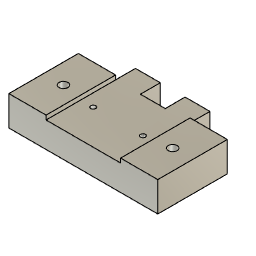
motor_mount_spacer_plate v51 (Autodesk Fusion 360 design; units mm, degrees)
Autodesk Fusion 360 part; units mm, degrees
sketch "Sketch1" plane through (0, 0, 0) normal (0, 0, 1) x (1, 0, 0)
  line L0 (0, 0) -> (57, 0)
  line L1 (57, 0) -> (57, 30)
  line L2 (57, 30) -> (0, 30)
  line L3 (0, 30) -> (0, 0)
  dimension "d1" = 57
  dimension "d2" = 30
  constraint horizontal L0
  constraint vertical L1
  constraint horizontal L2
  constraint vertical L3
  constraint coincident L0.start L3.end
  measures "d1" distance of L0.start L0.end
  measures "d2" distance of L0.start L2.end
extrude "Extrude1" add sketch "Sketch1" along normal blind 20.719
extrude "Extrude2" add 1 faces at (19, 20, 20.719) along direction (0, 0, 1) blind 10.719
extrude "Extrude3" add 1 faces at (19, 0, 10.4793) along direction (0, -1, 0) blind 10
extrude "Extrude4" cut 1 faces at (19, -10, 10.4793) along direction (0, 1, 0) blind 2
sketch "Sketch2" plane through (0, 0, 31.438) normal (0, 0, 1) x (-1, 0, 0)
  line L0 (0, 8) -> (-57, 8)
  line L1 (-57, 8) -> (-57, -30)
  line L2 (-57, -30) -> (0, -30)
  line L3 (0, -30) -> (0, 8)
  line L4 (0, -30) -> (0, -11)
  line L5 (0, -11) -> (-14.754, -11)
  line L6 (-57, -11) -> (-42.246, -11)
  dimension "d11" = 19
  dimension "d12" = 14.754
  dimension "d13" = 14.754
  constraint coincident L2.end L3.start
  constraint perpendicular L0 L4
  constraint perpendicular L4 L5
  constraint midpoint L1 L6.start
  constraint perpendicular L1 L6
  measures "d11" distance of L2.end L4.end
  measures "d12" distance of L4.end L5.end
  measures "d13" distance of L6.start L6.end
hole "Hole1" at (14.754, 11, 31.438) at (42.246, 11, 31.438) direction (0, 0, -1) diameter 6.6 depth 50 tip angle 180
sketch "Sketch3" plane through (0, 0, 31.438) normal (0, 0, 1) x (-1, 0, 0)
  circle A0 centre (-14.754, -11) radius 3.3
  circle A1 centre (-42.246, -11) radius 3.3
  line L0 (0, 8) -> (-57, 8)
  line L1 (-57, 8) -> (-57, -30)
  line L2 (-57, -30) -> (0, -30)
  line L3 (0, -30) -> (0, 8)
  line L4 (-14.754, -11) -> (-14.754, 0.251)
  line L5 (-42.246, -11) -> (-42.246, 0.251)
  dimension "d17" = 11.251
  dimension "d18" = 11.251
  constraint coincident A0.centre L4.start
  constraint vertical L4
  constraint coincident A1.centre L5.start
  constraint vertical L5
  measures "d17" distance of A0.centre L4.end
  measures "d18" distance of A1.centre L5.end
hole "Hole2" at (14.754, -0.251, 31.438) at (42.246, -0.251, 31.438) direction (0, 0, -1) diameter 6.6 depth 50 tip angle 180
delete_face "DeleteFace1" 1 faces at (15.0826, 7.7164, 20.9587)
delete_face "DeleteFace2" 1 faces at (42.5746, 7.7164, 20.9587)
delete_face "DeleteFace3" 1 faces at (15.0826, -3.5346, 20.9587)
delete_face "DeleteFace4" 1 faces at (42.5746, -3.5346, 20.9587)
sketch "Sketch4" plane through (0, 0, 31.438) normal (0, 0, 1) x (-1, 0, 0)
  line L0 (0, 8) -> (-57, 8)
  line L1 (-57, 8) -> (-57, -30)
  line L2 (-57, -30) -> (0, -30)
  line L3 (0, -30) -> (0, 8)
  line L4 (0, 8) -> (-14.754, 8)
  line L5 (-14.754, 8) -> (-14.754, -2)
  line L6 (-14.754, -2) -> (0, -2)
  line L7 (0, -2) -> (0, 8)
  line L8 (-57, 8) -> (-42.246, 8)
  line L9 (-42.246, 8) -> (-42.246, -2)
  line L10 (-42.246, -2) -> (-57, -2)
  line L11 (-57, -2) -> (-57, 8)
  dimension "d22" = 14.754
  dimension "d23" = 10
  dimension "d24" = 14.754
  dimension "d25" = 10
  constraint horizontal L4
  constraint vertical L5
  constraint horizontal L6
  constraint vertical L7
  constraint coincident L0.start L3.end
  constraint horizontal L8
  constraint vertical L9
  constraint horizontal L10
  constraint vertical L11
  constraint coincident L0.end L1.start
  measures "d22" distance of L0.start L4.end
  measures "d23" distance of L0.start L6.end
  measures "d24" distance of L0.end L8.end
  measures "d25" distance of L0.end L10.end
hole "Hole3" at (14.754, 2, 31.438) at (42.246, 2, 31.438) direction (0, 0, -1) diameter 6.6 depth 48 tip angle 180
delete_face "DeleteFace5" 1 faces at (15.0826, -1.2836, 20.9587)
delete_face "DeleteFace6" 1 faces at (42.5746, -1.2836, 20.9587)
sketch "Sketch5" plane through (0, 0, 31.438) normal (0, 0, 1) x (-1, 0, 0)
  line L0 (0, 8) -> (-57, 8)
  line L1 (-57, 8) -> (-57, -30)
  line L2 (-57, -30) -> (0, -30)
  line L3 (0, -30) -> (0, 8)
  line L4 (0, 8) -> (-28.5, 8)
  line L5 (-28.5, 8) -> (-28.5, -11)
  line L6 (-28.5, -11) -> (0, -11)
  line L7 (0, -11) -> (0, 8)
  line L8 (-28.5, -11) -> (-14.754, -11)
  line L9 (-14.754, -11) -> (-14.754, 2.746)
  line L10 (-14.754, 2.746) -> (-28.5, 2.746)
  line L11 (-28.5, 2.746) -> (-28.5, -11)
  line L12 (-14.754, 2.746) -> (-42.246, 2.746)
  line L13 (-42.246, 2.746) -> (-42.246, -24.746)
  line L14 (-42.246, -24.746) -> (-14.754, -24.746)
  line L15 (-14.754, -24.746) -> (-14.754, 2.746)
  dimension "d29" = 28.5
  dimension "d30" = 19
  dimension "d31" = 13.746
  dimension "d32" = 13.746
  dimension "d33" = 27.492
  dimension "d34" = 27.492
  constraint horizontal L4
  constraint vertical L5
  constraint horizontal L6
  constraint vertical L7
  constraint coincident L0.start L3.end
  constraint horizontal L8
  constraint vertical L9
  constraint horizontal L10
  constraint vertical L11
  constraint horizontal L12
  constraint vertical L13
  constraint horizontal L14
  constraint vertical L15
  measures "d29" distance of L0.start L4.end
  measures "d30" distance of L0.start L6.end
  measures "d31" distance of L5.end L8.end
  measures "d32" distance of L5.end L10.end
  measures "d33" distance of L9.end L12.end
  measures "d34" distance of L9.end L14.end
extrude "Extrude5" add 1 faces at (19, -8, 10.4793) along direction (0, -1, 0) blind 1
extrude "Extrude6" add 1 faces at (38, 30, 10.4793) along direction (0, 1, 0) blind 1
sketch "Sketch6" plane through (0, 0, 31.438) normal (0, 0, 1) x (-1, 0, 0)
  line L0 (-57, 9) -> (-57, -31)
  line L1 (-57, -31) -> (0, -31)
  line L2 (0, -31) -> (0, 9)
  line L3 (0, 9) -> (-57, 9)
  line L4 (0, -31) -> (-20, -31)
  line L5 (-20, -31) -> (-20, -41)
  line L6 (-20, -41) -> (0, -41)
  line L7 (0, -41) -> (0, -31)
  line L8 (-57, -31) -> (-37, -31)
  line L9 (-37, -31) -> (-37, -41)
  line L10 (-37, -41) -> (-57, -41)
  line L11 (-57, -41) -> (-57, -31)
  dimension "d42" = 20
  dimension "d43" = 10
  dimension "d44" = 20
  dimension "d45" = 10
  constraint horizontal L4
  constraint vertical L5
  constraint horizontal L6
  constraint vertical L7
  constraint coincident L1.end L2.start
  constraint horizontal L8
  constraint vertical L9
  constraint horizontal L10
  constraint vertical L11
  constraint coincident L0.end L1.start
  measures "d42" distance of L1.end L4.end
  measures "d43" distance of L1.end L6.end
  measures "d44" distance of L0.end L8.end
  measures "d45" distance of L0.end L10.end
extrude "Extrude7" add sketch "Sketch6" against normal up to surface (31.438 mm away) contours L1 L8 L9 L10 L11 | L1 L4 L5 L6 L7
extrude "Extrude8" add 2 faces at (13.3333, 41, 20.9587) (43.6667, 41, 20.9587) along direction (0, 1, 0) blind 10
extrude "Extrude9" cut 1 faces at (31.3333, 4.3333, 31.438) along direction (0, 0, -1) blind 5.719
extrude "Extrude10" add 1 faces at (0, 11, 17.146) along direction (-1, 0, 0) blind 1.25
extrude "Extrude11" add 1 faces at (57, 11, 17.146) along direction (1, 0, 0) blind 1.25
extrude "Extrude12" add 1 faces at (58.25, 11, 17.146) along direction (1, 0, 0) blind 0.25
extrude "Extrude13" add 1 faces at (-1.25, 11, 17.146) along direction (-1, 0, 0) blind 0.25
extrude "Extrude14" cut 1 faces at (20, 37.6667, 17.146) along direction (-1, 0, 0) blind 1.5
extrude "Extrude15" cut 1 faces at (37, 37.6667, 17.146) along direction (1, 0, 0) blind 1.5
sketch "Sketch8" plane through (0, 0, 25.719) normal (0, 0, 1) x (-1, 0, 0)
  line L0 (-38.5, -51) -> (-38.5, -31)
  line L1 (-38.5, -31) -> (-18.5, -31)
  line L2 (-18.5, -31) -> (-18.5, -51)
  line L3 (-18.5, -51) -> (1.5, -51)
  line L4 (1.5, -51) -> (1.5, 9)
  line L5 (1.5, 9) -> (-58.5, 9)
  line L6 (-58.5, 9) -> (-58.5, -51)
  line L7 (-58.5, -51) -> (-38.5, -51)
  line L8 (-28.5, -31) -> (-28.5, -11)
  line L9 (-28.5, -11) -> (-13.5, -11)
  line L10 (-13.5, -11) -> (-13.5, 4)
  line L11 (-13.5, 4) -> (-28.5, 4)
  line L12 (-28.5, 4) -> (-28.5, -11)
  line L13 (-13.5, 4) -> (-43.5, 4)
  line L14 (-43.5, 4) -> (-43.5, -26)
  line L15 (-43.5, -26) -> (-13.5, -26)
  line L16 (-13.5, -26) -> (-13.5, 4)
  dimension "d64" = 15
  dimension "d65" = 15
  dimension "d66" = 30
  dimension "d67" = 30
  constraint midpoint L1 L8.start
  constraint perpendicular L5 L8
  constraint horizontal L9
  constraint vertical L10
  constraint horizontal L11
  constraint vertical L12
  constraint horizontal L13
  constraint vertical L14
  constraint horizontal L15
  constraint vertical L16
  measures "d64" distance of L8.end L9.end
  measures "d65" distance of L8.end L11.end
  measures "d66" distance of L10.end L13.end
  measures "d67" distance of L10.end L15.end
extrude "Extrude16" add 1 faces at (38.5, -9, 8.573) along direction (0, -1, 0) blind 5
extrude "Extrude17" add 2 faces at (11.8333, 51, 17.146) (45.1667, 51, 17.146) along direction (0, 1, 0) blind 5.688
extrude "Extrude18" add 1 faces at (25.1667, 31, 8.573) along direction (0, 1, 0) blind 0.688
extrude "Extrude19" cut 1 faces at (38.5, -14, 8.573) along direction (0, 1, 0) blind 0.788
extrude "Extrude20" add 1 faces at (38.5, -13.212, 8.573) along direction (0, -1, 0) blind 0.1
extrude "Extrude21" cut 1 faces at (18.5, 40.0213, 17.146) along direction (-1, 0, 0) blind 2.5
extrude "Extrude22" cut 1 faces at (38.5, 40.0213, 17.146) along direction (1, 0, 0) blind 2.5
extrude "Extrude23" cut 1 faces at (10.1667, 56.688, 17.146) along direction (0, -1, 0) blind 3
extrude "Extrude24" cut 1 faces at (46.8333, 56.688, 17.146) along direction (0, -1, 0) blind 3
sketch "Sketch9" plane through (0, 0, 25.719) normal (0, 0, 1) x (-1, 0, 0)
  line L0 (-58.5, -53.688) -> (-41, -53.688)
  line L1 (-41, -53.688) -> (-41, -31.688)
  line L2 (-41, -31.688) -> (-16, -31.688)
  line L3 (-16, -31.688) -> (-16, -53.688)
  line L4 (-16, -53.688) -> (1.5, -53.688)
  line L5 (1.5, -53.688) -> (1.5, 13.312)
  line L6 (1.5, 13.312) -> (-58.5, 13.312)
  line L7 (-58.5, 13.312) -> (-58.5, -53.688)
  line L8 (-43.5, -26) -> (-43.5, -23)
  line L9 (-43.5, -23) -> (-13.5, -23)
  line L10 (-13.5, -23) -> (-13.5, 7)
  line L11 (-13.5, 7) -> (-43.5, 7)
  line L12 (-43.5, 7) -> (-43.5, -23)
  dimension "d89" = 3
  dimension "d90" = 30
  dimension "d91" = 30
  constraint vertical L8
  constraint horizontal L9
  constraint vertical L10
  constraint horizontal L11
  constraint vertical L12
  measures "d89" distance of L8.start L8.end
  measures "d90" distance of L8.end L9.end
  measures "d91" distance of L8.end L11.end
sketch "Sketch10" plane through (0, 0, 25.719) normal (0, 0, 1) x (-1, 0, 0)
  line L0 (-58.5, -53.688) -> (-41, -53.688)
  line L1 (-41, -53.688) -> (-41, -31.688)
  line L2 (-41, -31.688) -> (-16, -31.688)
  line L3 (-16, -31.688) -> (-16, -53.688)
  line L4 (-16, -53.688) -> (1.5, -53.688)
  line L5 (1.5, -53.688) -> (1.5, 13.312)
  line L6 (1.5, 13.312) -> (-58.5, 13.312)
  line L7 (-58.5, 13.312) -> (-58.5, -53.688)
  line L8 (-43.5, 7) -> (-43.5, 6.312)
  line L9 (-43.5, 6.312) -> (-13.5, 6.312)
  line L10 (-13.5, 6.312) -> (-13.5, -23.688)
  line L11 (-13.5, -23.688) -> (-43.5, -23.688)
  line L12 (-43.5, -23.688) -> (-43.5, 6.312)
  dimension "d95" = 0.688
  dimension "d96" = 30
  dimension "d97" = 30
  constraint vertical L8
  constraint horizontal L9
  constraint vertical L10
  constraint horizontal L11
  constraint vertical L12
  measures "d95" distance of L8.start L8.end
  measures "d96" distance of L8.end L9.end
  measures "d97" distance of L8.end L11.end
sketch "Sketch11" plane through (0, 0, 25.719) normal (0, 0, 1) x (-1, 0, 0)
  line L0 (-58.5, -53.688) -> (-41, -53.688)
  line L1 (-41, -53.688) -> (-41, -31.688)
  line L2 (-41, -31.688) -> (-16, -31.688)
  line L3 (-16, -31.688) -> (-16, -53.688)
  line L4 (-16, -53.688) -> (1.5, -53.688)
  line L5 (1.5, -53.688) -> (1.5, 13.312)
  line L6 (1.5, 13.312) -> (-58.5, 13.312)
  line L7 (-58.5, 13.312) -> (-58.5, -53.688)
  line L8 (-13.5, 6.312) -> (-13.5, 8.624)
  line L9 (-13.5, 8.624) -> (-43.5, 8.624)
  line L10 (-43.5, 8.624) -> (-43.5, -21.376)
  line L11 (-43.5, -21.376) -> (-13.5, -21.376)
  line L12 (-13.5, -21.376) -> (-13.5, 8.624)
  dimension "d101" = 2.312
  dimension "d102" = 30
  dimension "d103" = 30
  constraint vertical L8
  constraint horizontal L9
  constraint vertical L10
  constraint horizontal L11
  constraint vertical L12
  measures "d101" distance of L8.start L8.end
  measures "d102" distance of L8.end L9.end
  measures "d103" distance of L8.end L11.end
extrude "Extrude25" cut 2 faces at (10.1667, 53.688, 17.146) (46.8333, 53.688, 17.146) along direction (0, -1, 0) blind 2
extrude "Extrude26" cut 2 faces at (10.1667, 51.688, 17.146) (46.8333, 51.688, 17.146) along direction (0, -1, 0) blind 2
extrude "Extrude27" add 1 faces at (38.5, -13.312, 8.573) along direction (0, -1, 0) blind 5
extrude "Extrude28" cut 2 faces at (46.8333, 49.688, 17.146) (10.1667, 49.688, 17.146) along direction (0, -1, 0) blind 1.256
extrude "Extrude29" cut 1 faces at (32.6667, 31.688, 17.146) along direction (0, -1, 0) blind 1.256
extrude "Extrude30" add 1 faces at (38.5, -18.312, 8.573) along direction (0, -1, 0) blind 1.256
extrude "Extrude31" cut 1 faces at (38.5, -19.568, 8.573) along direction (0, 1, 0) blind 3
sketch "Sketch12" plane through (0, 0, 25.719) normal (0, 0, 1) x (-1, 0, 0)
  line L0 (1.5, 16.568) -> (-58.5, 16.568)
  line L1 (-58.5, 16.568) -> (-58.5, -48.432)
  line L2 (-58.5, -48.432) -> (-41, -48.432)
  line L3 (-41, -48.432) -> (-41, -30.432)
  line L4 (-41, -30.432) -> (-16, -30.432)
  line L5 (-16, -30.432) -> (-16, -48.432)
  line L6 (-16, -48.432) -> (1.5, -48.432)
  line L7 (1.5, -48.432) -> (1.5, 16.568)
  line L8 (-43.5, -21.376) -> (-43.5, -18.432)
  line L9 (-43.5, -18.432) -> (-13.5, -18.432)
  line L10 (-13.5, -18.432) -> (-13.5, 11.568)
  line L11 (-13.5, 11.568) -> (-43.5, 11.568)
  line L12 (-43.5, 11.568) -> (-43.5, -18.432)
  dimension "d121" = 2.944
  dimension "d122" = 30
  dimension "d123" = 30
  constraint vertical L8
  constraint horizontal L9
  constraint vertical L10
  constraint horizontal L11
  constraint vertical L12
  measures "d121" distance of L8.start L8.end
  measures "d122" distance of L8.end L9.end
  measures "d123" distance of L8.end L11.end
hole "Hole9" at (13.5, 18.432, 25.719) at (13.5, -11.568, 25.719) at (43.5, -11.568, 25.719) at (43.5, 18.432, 25.719) direction (0, 0, -1) diameter 6.6 depth 36 tip angle 180
sketch "Sketch13" plane through (0, 0, 25.719) normal (0, 0, 1) x (-1, 0, 0)
  circle A0 centre (-43.5, 11.568) radius 3.3
  circle A1 centre (-13.5, -18.432) radius 3.3
  circle A2 centre (-13.5, 11.568) radius 3.3
  circle A3 centre (-43.5, -18.432) radius 3.3
  line L0 (1.5, 16.568) -> (-58.5, 16.568)
  line L1 (-58.5, 16.568) -> (-58.5, -48.432)
  line L2 (-58.5, -48.432) -> (-41, -48.432)
  line L3 (-41, -48.432) -> (-41, -30.432)
  line L4 (-41, -30.432) -> (-16, -30.432)
  line L5 (-16, -30.432) -> (-16, -48.432)
  line L6 (-16, -48.432) -> (1.5, -48.432)
  line L7 (1.5, -48.432) -> (1.5, 16.568)
  line L8 (-43.5, 11.568) -> (-43.5, -3.432)
  line L9 (-13.5, 11.568) -> (-13.5, -3.432)
  dimension "d127" = 15
  dimension "d128" = 15
  constraint coincident A0.centre L8.start
  constraint vertical L8
  constraint coincident A2.centre L9.start
  constraint vertical L9
  measures "d127" distance of A0.centre L8.end
  measures "d128" distance of A2.centre L9.end
hole "Hole10" at (13.5, 3.432, 25.719) at (43.5, 3.432, 25.719) direction (0, 0, -1) diameter 6.6 depth 48 tip angle 180
delete_face "DeleteFace7" 1 faces at (43.8286, -14.8516, 17.146)
delete_face "DeleteFace8" 1 faces at (13.6645, -14.8639, 8.573)
extrude "Extrude32" add 1 faces at (58.5, 5.0987, 8.573) along direction (1, 0, 0) blind 45
extrude "Extrude33" add 1 faces at (-1.5, 5.0987, 8.573) along direction (-1, 0, 0) blind 45
extrude "Extrude34" add 1 faces at (3.5, -16.568, 17.146) along direction (0, -1, 0) blind 5
delete_face "DeleteFace9" 1 faces at (13.6645, 15.1361, 8.573)
delete_face "DeleteFace10" 1 faces at (43.8286, 15.1484, 17.146)
sketch "Sketch14" plane through (0, 0, 25.719) normal (0, 0, 1) x (-1, 0, 0)
  circle A0 centre (-13.5, -3.432) radius 3.3
  circle A1 centre (-43.5, -3.432) radius 3.3
  line L0 (-103.5, 21.568) -> (-103.5, -48.432)
  line L1 (-103.5, -48.432) -> (-41, -48.432)
  line L2 (-41, -48.432) -> (-41, -30.432)
  line L3 (-41, -30.432) -> (-16, -30.432)
  line L4 (-16, -30.432) -> (-16, -48.432)
  line L5 (-16, -48.432) -> (46.5, -48.432)
  line L6 (46.5, -48.432) -> (46.5, 21.568)
  line L7 (46.5, 21.568) -> (-103.5, 21.568)
  line L8 (-16, -30.432) -> (34, -30.432)
  line L9 (34, -30.432) -> (21.5, -30.432)
  line L10 (21.5, -30.432) -> (46.5, -30.432)
  line L11 (46.5, -30.432) -> (46.5, -48.432)
  line L12 (46.5, -48.432) -> (21.5, -48.432)
  line L13 (21.5, -48.432) -> (21.5, -30.432)
  line L14 (-41, -30.432) -> (-78.5, -30.432)
  line L15 (-78.5, -30.432) -> (-103.5, -30.432)
  line L16 (-103.5, -30.432) -> (-103.5, -48.432)
  line L17 (-103.5, -48.432) -> (-78.5, -48.432)
  line L18 (-78.5, -48.432) -> (-78.5, -30.432)
  dimension "d138" = 50
  dimension "d139" = 12.5
  dimension "d140" = 37.5
  constraint coincident L3.end L4.start
  constraint perpendicular L4 L8
  constraint perpendicular L6 L9
  constraint horizontal L10
  constraint vertical L11
  constraint horizontal L12
  constraint vertical L13
  constraint coincident L5.end L6.start
  constraint coincident L2.end L3.start
  constraint perpendicular L2 L14
  constraint horizontal L15
  constraint vertical L16
  constraint horizontal L17
  constraint vertical L18
  constraint coincident L0.end L1.start
  measures "d138" distance of L3.end L8.end
  measures "d139" distance of L8.end L9.end
  measures "d140" distance of L2.end L14.end
extrude "Extrude35" cut sketch "Sketch14" against normal blind 30 contours L0 L1 L15 L16 L17 L18 | L5 L6 L8 L9 L10 L11 L12 L13
sketch "Sketch15" plane through (0, 0, 25.719) normal (0, 0, 1) x (-1, 0, 0)
  circle A0 centre (-43.5, -3.432) radius 3.3
  circle A1 centre (-13.5, -3.432) radius 3.3
  line L0 (21.5, -48.432) -> (21.5, -30.432)
  line L1 (21.5, -30.432) -> (46.5, -30.432)
  line L2 (46.5, -30.432) -> (46.5, 21.568)
  line L3 (46.5, 21.568) -> (-103.5, 21.568)
  line L4 (-103.5, 21.568) -> (-103.5, -30.432)
  line L5 (-103.5, -30.432) -> (-78.5, -30.432)
  line L6 (-78.5, -30.432) -> (-78.5, -48.432)
  line L7 (-78.5, -48.432) -> (-41, -48.432)
  line L8 (-41, -48.432) -> (-41, -30.432)
  line L9 (-41, -30.432) -> (-16, -30.432)
  line L10 (-16, -30.432) -> (-16, -48.432)
  line L11 (-16, -48.432) -> (21.5, -48.432)
  line L12 (21.5, -39.432) -> (9, -39.432)
  line L13 (9, -39.432) -> (21.5, -39.432)
  line L14 (21.5, -39.432) -> (21.5, -30.432)
  line L15 (21.5, -30.432) -> (9, -30.432)
  line L16 (9, -30.432) -> (9, -39.432)
  line L17 (9, -30.432) -> (21.5, -30.432)
  line L18 (21.5, -30.432) -> (21.5, -48.432)
  line L19 (21.5, -48.432) -> (9, -48.432)
  line L20 (9, -48.432) -> (9, -30.432)
  line L21 (-78.5, -39.432) -> (-66, -39.432)
  line L22 (-66, -39.432) -> (-78.5, -39.432)
  line L23 (-78.5, -39.432) -> (-78.5, -30.432)
  line L24 (-78.5, -30.432) -> (-66, -30.432)
  line L25 (-66, -30.432) -> (-66, -39.432)
  line L26 (-66, -39.432) -> (-78.5, -39.432)
  line L27 (-78.5, -39.432) -> (-78.5, -48.432)
  line L28 (-78.5, -48.432) -> (-66, -48.432)
  line L29 (-66, -48.432) -> (-66, -39.432)
  dimension "d143" = 12.5
  dimension "d144" = 12.5
  constraint midpoint L0 L12.start
  constraint perpendicular L2 L12
  constraint horizontal L13
  constraint vertical L14
  constraint horizontal L15
  constraint vertical L16
  constraint coincident L0.end L1.start
  constraint horizontal L17
  constraint vertical L18
  constraint horizontal L19
  constraint vertical L20
  constraint coincident L0.start L11.end
  constraint midpoint L6 L21.start
  constraint perpendicular L6 L21
  constraint horizontal L22
  constraint vertical L23
  constraint horizontal L24
  constraint vertical L25
  constraint coincident L5.end L6.start
  constraint horizontal L26
  constraint vertical L27
  constraint horizontal L28
  constraint vertical L29
  constraint coincident L6.end L7.start
  measures "d143" distance of L12.start L12.end
  measures "d144" distance of L21.start L21.end
extrude "Extrude36" cut sketch "Sketch15" against normal blind 90 contours L0 L11 L12 L13 L18 L19 L20 | L0 L12 L13 L14 L15 L16 L17 L18 L20 | L6 L7 L21 L22 L26 L27 L28 L29 | L6 L21 L22 L23 L24 L25 L26
sketch "Sketch16" plane through (0, 0, 25.719) normal (0, 0, 1) x (-1, 0, 0)
  line L0 (9, -30.432) -> (46.5, -30.432)
  line L1 (46.5, -30.432) -> (46.5, 21.568)
  line L2 (46.5, 21.568) -> (-103.5, 21.568)
  line L3 (-103.5, 21.568) -> (-103.5, -30.432)
  line L4 (-103.5, -30.432) -> (-66, -30.432)
  line L5 (-66, -30.432) -> (-66, -48.432)
  line L6 (-66, -48.432) -> (-41, -48.432)
  line L7 (-41, -48.432) -> (-41, -30.432)
  line L8 (-41, -30.432) -> (-16, -30.432)
  line L9 (-16, -30.432) -> (-16, -48.432)
  line L10 (-16, -48.432) -> (9, -48.432)
  line L11 (9, -48.432) -> (9, -30.432)
  circle A0 centre (-43.5, -3.432) radius 3.3
  circle A1 centre (-13.5, -3.432) radius 3.3
  line L12 (-53.5, -48.432) -> (-53.5, -13.432)
  line L13 (-3.5, -48.432) -> (-3.5, -13.432)
  dimension "d147" = 35
  dimension "d148" = 35
  constraint midpoint L6 L12.start
  constraint perpendicular L6 L12
  constraint midpoint L10 L13.start
  constraint perpendicular L10 L13
  measures "d147" distance of L12.start L12.end
  measures "d148" distance of L13.start L13.end
delete_face "DeleteFace11" 1 faces at (43.8286, 0.1484, 17.146)
delete_face "DeleteFace12" 1 faces at (13.6645, 0.1361, 8.573)
hole "Hole11" at (3.5, 13.432, 25.719) at (53.5, 13.432, 25.719) direction (0, 0, -1) diameter 6.6 depth 45 tip angle 180
sketch "Sketch17" plane through (0, 0, 25.719) normal (0, 0, 1) x (-1, 0, 0)
  circle A0 centre (-3.5, -13.432) radius 3.3
  circle A1 centre (-53.5, -13.432) radius 3.3
  line L0 (9, -30.432) -> (46.5, -30.432)
  line L1 (46.5, -30.432) -> (46.5, 21.568)
  line L2 (46.5, 21.568) -> (-103.5, 21.568)
  line L3 (-103.5, 21.568) -> (-103.5, -30.432)
  line L4 (-103.5, -30.432) -> (-66, -30.432)
  line L5 (-66, -30.432) -> (-66, -48.432)
  line L6 (-66, -48.432) -> (-41, -48.432)
  line L7 (-41, -48.432) -> (-41, -30.432)
  line L8 (-41, -30.432) -> (-16, -30.432)
  line L9 (-16, -30.432) -> (-16, -48.432)
  line L10 (-16, -48.432) -> (9, -48.432)
  line L11 (9, -48.432) -> (9, -30.432)
  line L12 (-3.5, -13.432) -> (-3.5, 6.568)
  line L13 (-53.5, -13.432) -> (-53.5, 6.568)
  dimension "d152" = 20
  dimension "d153" = 20
  constraint coincident A0.centre L12.start
  constraint vertical L12
  constraint coincident A1.centre L13.start
  constraint vertical L13
  measures "d152" distance of A0.centre L12.end
  measures "d153" distance of A1.centre L13.end
hole "Hole12" at (3.5, -6.568, 25.719) at (53.5, -6.568, 25.719) direction (0, 0, -1) diameter 5.035 depth 20 tip angle 180
thread "Thread1" "ISO Metric profile 6.0 M6x1 6H"
delete_face "DeleteFace13" 1 faces at (53.8286, 10.1484, 17.146)
delete_face "DeleteFace14" 1 faces at (3.6645, 10.1361, 8.573)
extrude "Extrude37" add 1 faces at (3.5, -21.568, 17.146) along direction (0, -1, 0) blind 20
extrude "Extrude38" cut 3 faces at (78.5, 30.432, 17.146) (32.6667, 30.432, 17.146) (-21.5, 30.432, 17.146) along direction (0, -1, 0) blind 2
sketch "Sketch18" plane through (0, 0, 25.719) normal (0, 0, 1) x (-1, 0, 0)
  circle A0 centre (-53.5, 6.568) radius 2.5175
  circle A1 centre (-3.5, 6.568) radius 2.5175
  line L0 (-41, -48.432) -> (-41, -28.432)
  line L1 (-41, -28.432) -> (-16, -28.432)
  line L2 (-16, -28.432) -> (-16, -48.432)
  line L3 (-16, -48.432) -> (9, -48.432)
  line L4 (9, -48.432) -> (9, -28.432)
  line L5 (9, -28.432) -> (46.5, -28.432)
  line L6 (46.5, -28.432) -> (46.5, 41.568)
  line L7 (46.5, 41.568) -> (-103.5, 41.568)
  line L8 (-103.5, 41.568) -> (-103.5, -28.432)
  line L9 (-103.5, -28.432) -> (-66, -28.432)
  line L10 (-66, -28.432) -> (-66, -48.432)
  line L11 (-66, -48.432) -> (-41, -48.432)
  line L12 (-103.5, 6.568) -> (-83.5, 6.568)
  line L13 (46.5, 6.568) -> (26.5, 6.568)
  dimension "d161" = 20
  dimension "d162" = 20
  constraint midpoint L8 L12.start
  constraint perpendicular L8 L12
  constraint midpoint L6 L13.start
  constraint perpendicular L6 L13
  measures "d161" distance of L12.start L12.end
  measures "d162" distance of L13.start L13.end
hole "Hole13" at (-26.5, -6.568, 25.719) at (83.5, -6.568, 25.719) direction (0, 0, -1) diameter 9 depth 45 tip angle 180
sketch "Sketch19" plane through (0, 0, 25.719) normal (0, 0, 1) x (-1, 0, 0)
  circle A0 centre (26.5, 6.568) radius 4.5
  circle A1 centre (-83.5, 6.568) radius 4.5
  circle A2 centre (-53.5, 6.568) radius 2.5175
  circle A3 centre (-3.5, 6.568) radius 2.5175
  line L0 (-41, -48.432) -> (-41, -28.432)
  line L1 (-41, -28.432) -> (-16, -28.432)
  line L2 (-16, -28.432) -> (-16, -48.432)
  line L3 (-16, -48.432) -> (9, -48.432)
  line L4 (9, -48.432) -> (9, -28.432)
  line L5 (9, -28.432) -> (46.5, -28.432)
  line L6 (46.5, -28.432) -> (46.5, 41.568)
  line L7 (46.5, 41.568) -> (-103.5, 41.568)
  line L8 (-103.5, 41.568) -> (-103.5, -28.432)
  line L9 (-103.5, -28.432) -> (-66, -28.432)
  line L10 (-66, -28.432) -> (-66, -48.432)
  line L11 (-66, -48.432) -> (-41, -48.432)
  line L12 (-66, -28.432) -> (-103.5, -28.432)
  line L13 (-103.5, -28.432) -> (-103.5, 41.568)
  line L14 (-103.5, 41.568) -> (-66, 41.568)
  line L15 (-66, 41.568) -> (-66, -28.432)
  line L16 (9, -28.432) -> (46.5, -28.432)
  line L17 (46.5, -28.432) -> (46.5, 41.568)
  line L18 (46.5, 41.568) -> (9, 41.568)
  line L19 (9, 41.568) -> (9, -28.432)
  constraint horizontal L12
  constraint vertical L13
  constraint horizontal L14
  constraint vertical L15
  constraint coincident L7.end L8.start
  constraint coincident L9.end L10.start
  constraint horizontal L16
  constraint vertical L17
  constraint horizontal L18
  constraint vertical L19
  constraint coincident L6.end L7.start
  constraint coincident L4.end L5.start
extrude "Extrude39" add sketch "Sketch19" along normal blind 4.281 contours L7 L8 L9 L12 L13 L14 L15 | L5 L6 L7 L16 L17 L18 L19
equation "d11 = ( 38.000 / 2 ) * 1 mm"
equation "d29 = ( 57.000 / 2 ) * 1 mm"
equation "d30 = ( 38.000 / 2 ) * 1 mm"
equation "d31 = ( 27.492 / 2 ) * 1 mm"
equation "d32 = ( 27.492 / 2 ) * 1 mm"
equation "d166 = 5 mm - 0.719 mm"
